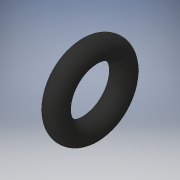
# Autodesk Inventor part: High-Temperature Silicone O-Ring(1283N198)
Saved by Autodesk Inventor 2018 (Build 220112000, 112)
## iProperties
Created: 2020-03-27
Part Number: High-Temperature Silicone O-Ring(1283N198)
Material: Generic
Document SubType Name: Modeling
Designer: emile
Density: 1 g/cm^3
Appearance: Rubber - Black
Author: emile
Autodesk Inventor part; units mm, degrees
ref_plane "YZ Plane" through (0, 0, 0) normal (1, 0, 0) x (0, 1, 0)
ref_plane "XZ Plane" through (0, 0, 0) normal (0, 1, 0) x (-1, 0, 0)
ref_plane "XY Plane" through (0, 0, 0) normal (0, 0, 1) x (1, 0, 0)
sketch "Sketch1" plane through (0, 0, 0) normal (0, 1, 0) x (-1, 0, 0)
  circle A0 centre (0, -5.734) radius 1.7653
  line L0 (0, -5.734) -> (0, -3.9688) construction
  line L1 (2.4714, 0) -> (-2.4714, 0) projected
  point P0 (0, 0)
  dimension "d1" = 3.5306
  dimension "d2" = 3.9688
  constraints: 2 end point, 2 vertical alignment, 1 vertical, 2 other
  measures "d2" distance of point (0, 0) L0.end
revolve "Revolution1" add sketch "Sketch1" angle 360 about axis through (-10, 0, 0) along (1, 0, 0)
body "Solid1"
